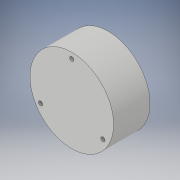
# Autodesk Inventor part: 볼캐스터 받침
Saved by Autodesk Inventor 2019.5 (Build 235369000, 369)
## iProperties
Created: 2021-08-25
Part Number: 볼캐스터 받침
Material: 일반
Document SubType Name: Modeling
Designer: msj19
Density: 1 g/cm^3
Appearance: 기본값
Author: msj19
Autodesk Inventor part; units mm, degrees
ref_plane "우측면도" through (0, 0, 0) normal (1, 0, 0) x (0, 1, 0)
ref_plane "평면도" through (0, 0, 0) normal (0, 1, 0) x (-1, 0, 0)
ref_plane "정면도" through (0, 0, 0) normal (0, 0, 1) x (1, 0, 0)
sketch "스케치2" plane through (0, 0, 0) normal (0, 0, 1) x (1, 0, 0)
  circle A0 centre (0, 0) radius 28
  circle A1 centre (0, 0) radius 32.5
  circle A2 centre (0, 28) radius 1.625 construction
  circle A3 centre (-24.2487, -14) radius 1.625 construction
  circle A4 centre (24.2487, -14) radius 1.625 construction
  line L0 (0, 28) -> (0, 0) construction
  dimension "d8" = 56
  dimension "d9" = 65
  dimension "d10" = 3.25
  dimension "d13" = 360
  constraints: 4 centre point, 2 coincident, 2 end point, 1 vertical, 1 vertical alignment, 9 other
  measures "d9" diameter of A1
  measures "d10" diameter of A2
extrude "돌출1" add sketch "스케치2" along normal blind 28.3 contours A0 | A1
sketch "스케치3" plane through (0, 0, 28.3) normal (0, 0, 1) x (1, 0, 0)
  circle A0 centre (0, 28) radius 1.625 projected
  circle A1 centre (24.2487, -14) radius 1.625 projected
  circle A2 centre (-24.2487, -14) radius 1.625 projected
  point P0 (0, 0)
extrude "돌출2" cut sketch "스케치3" against normal blind 100
